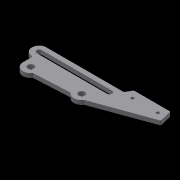
# Autodesk Inventor part: ForearmLeftEnd
Saved by Autodesk Inventor 2015 (Build 190159000, 159)
## iProperties
Created: 2014-10-05
Part Number: ForearmLeftEnd
Material: Generic
Document SubType Name: Modeling
Designer: Val
Density: 1 g/cm^3
Appearance: Default
Mass: 9.61038 g
Surface Area: 67.6636 cm^2
Volume: 9.61038 cm^3
Author: Val
Autodesk Inventor part; units mm, degrees
ref_plane "YZ Plane" through (0, 0, 0) normal (1, 0, 0) x (0, 1, 0)
ref_plane "XZ Plane" through (0, 0, 0) normal (0, 1, 0) x (-1, 0, 0)
ref_plane "XY Plane" through (0, 0, 0) normal (0, 0, 1) x (1, 0, 0)
sketch "Base" plane through (0, 0, 0) normal (0, 0, 1) x (1, 0, 0)
  arc A0 (-53.9833, -2.5) -> (-40.2726, -6.1797) centre (-46.5, -2) ccw
  line L0 (-6.0829, -4.3873) -> (-40.2726, -6.1797)
  arc A1 (-6.0829, -4.3873) -> (6.3177, -4.0419) centre (0, 0) ccw
  line L1 (60.0086, 15.5) -> (6.3177, -4.0419)
  circle A2 centre (52, 20.5) radius 1.5 construction
  circle A3 centre (28, 20.5) radius 1.5 construction
  line L2 (57.0167, 27.5) -> (60.0086, 15.5)
  line L3 (57.0167, 27.5) -> (-53.9833, 27.5)
  line L4 (-53.9833, -2.5) -> (-53.9833, 27.5)
  line L5 (52, 20.5) -> (28, 20.5) construction
  dimension "d3" = 24
  dimension "d4" = 3
  dimension "d7" = 104
  dimension "d16" = 20
  dimension "d17" = 111
  dimension "d19" = 30
  dimension "d22" = 86.999
  dimension "d25" = 28
  dimension "d26" = 7.5
  dimension "d31" = 27.5
  dimension "d32" = 12
  dimension "d45" = 46.5
  dimension "d46" = 2
  dimension "d47" = 4.5
  dimension "d64" = 7
  constraints: 12 end point, 4 centre point, 4 point on circle, 2 equal radius, 2 horizontal, 1 coincident, 1 vertical
  measures "d3" distance of L5.end L5.start
  measures "d4" diameter of A2
  measures "d7" angle of L3 L2
  measures "d16" angle of L1 L3
  measures "d17" distance of L2.start L3.end
  measures "d19" distance of L4.start L3.end
  measures "d22" angle of L0 L4
  measures "d25" horizontal distance of A1.centre L5.end
  measures "d26" radius of A1
  measures "d31" distance from line of L3 A1.centre
  measures "d32" vertical distance of L2.start L1.start
  measures "d45" horizontal distance of A0.centre A1.centre
  measures "d46" vertical distance of A1.centre A0.centre
  measures "d47" distance from line of L0 A0.centre
  measures "d64" distance between parallel lines of L3 L5
extrude "BaseFeature" add sketch "Base" along normal blind 4
fillet "EndFilletsFeature" radius 1 2 edges at (60.0086, 15.5, 2) (57.0167, 27.5, 2)
sketch "BaseMountHoles" plane through (0, 0, 0) normal (0, 0, -1) x (-1, 0, 0)
  arc A0 (40.2726, -6.1797) -> (53.9833, -2.5) centre (46.5, -2) ccw projected
  point P0 (0, 0)
hole "BaseMountHolesFeature" at (-46.5, -2, 0) at (0, 0, 0) direction (0, 0, 1) diameter 6 end through all
sketch "CuffMountHoles" plane through (0, 0, 0) normal (0, 0, -1) x (-1, 0, 0)
  circle A0 centre (-52, 20.5) radius 1.5 construction
  circle A1 centre (-28, 20.5) radius 1.5 construction
  point P0 (0, 0)
hole "CuffMountHolesFeature" at (52, 20.5, 0) at (28, 20.5, 0) direction (0, 0, 1) diameter 3 end through all
sketch "ExternalAssemblyGeometry" plane through (0, 0, 4) normal (0, 0, 1) x (1, 0, 0)
  circle A0 centre (-4.2211, 14.5) radius 2.4585 construction
  circle A1 centre (-12.2211, 14.5) radius 2.4585 construction
  circle A2 centre (-33.6105, 14.5) radius 2.4585 construction
  circle A3 centre (-55, 14.5) radius 2.4585 construction
  line L0 (16.9953, 21.5) -> (-152.0047, 21.5) construction
  line L1 (-55, 14.5) -> (12, 14.5) construction
  circle A4 centre (-55, 14.5) radius 7
  line L2 (-53.9833, 27.5) -> (56.2354, 27.5) projected
  line L3 (-53.9833, -2.5) -> (-53.9833, 27.5) projected
  dimension "d57" = 67
  dimension "d72" = 14
  dimension "d73" = 6
  dimension "d74" = 169
  dimension "d75" = 4.917
  dimension "d76" = 8
  dimension "d77" = 1.0167
  dimension "d78" = 21.3895
  dimension "d79" = 21.3895
  dimension "d80" = 70.9786
  constraints: 5 centre point, 4 end point, 3 equal radius, 3 point on line, 1 coincident, 1 horizontal, 1 tangent
  measures "d57" distance of L1.start L1.end
  measures "d72" diameter of A4
  measures "d73" distance between parallel lines of L2 L0
  measures "d74" distance of L0.start L0.end
  measures "d75" diameter of A0
  measures "d76" distance of A1.centre A0.centre
  measures "d77" distance from line of L1.start L3
  measures "d78" distance of L1.start A2.centre
  measures "d79" distance of A2.centre A1.centre
  measures "d80" distance from line of L0.start L3
extrude "MountRailEndFeature" add sketch "ExternalAssemblyGeometry" against normal up to surface (4 mm away)
sketch "MountRail" plane through (0, 0, 0) normal (0, 0, -1) x (-1, 0, 0)
  line L0 (55, 14.5) -> (-12, 14.5) construction
  circle A0 centre (55, 14.5) radius 2.4585 construction
  circle A1 centre (-12, 14.5) radius 2.4585
  circle A2 centre (55, 14.5) radius 2.4585
  line L1 (55, 12.0415) -> (-12, 12.0415)
  line L2 (55, 16.9585) -> (-12, 16.9585)
  point P0 (0, 0)
  constraints: 6 point on circle, 4 end point, 4 tangent, 2 centre point, 2 coincident, 2 equal radius
extrude "MountRailFeature" cut sketch "MountRail" against normal through all
sketch "TopAngleCut" plane through (0, 0, 0) normal (0, 0, -1) x (-1, 0, 0)
  line L0 (53.9833, 27.5) -> (-56.2354, 27.5) construction
  line L1 (-22.2354, 27.5) -> (-18.7284, 21.4258)
  line L2 (53.9833, 21.4258) -> (-18.7284, 21.4258)
  line L3 (-22.2354, 27.5) -> (53.9833, 27.5)
  line L4 (53.9833, 21.4258) -> (53.9833, 27.5)
  line L5 (53.9833, 21.4258) -> (53.9833, 27.5) projected
  point P0 (0, 0)
  point P1 (-57.0167, 27.5)
  dimension "d65" = 120
  dimension "d66" = 34
  constraints: 8 end point, 2 horizontal, 1 collinear, 1 point on line
  measures "d65" angle of L1 L2
  measures "d66" distance of L0.end L1.start
extrude "TopAngleCutFeature" cut sketch "TopAngleCut" against normal through all
fillet "TopAngleCutFilletsFeature" radius 1 2 edges at (22.2354, 27.5, 2) (18.7284, 21.4258, 2)
fillet "BodyFilletFeature" radius 1 2 edges at (-53.9833, 21.4258, 2) (-53.9833, 7.5742, 2)
